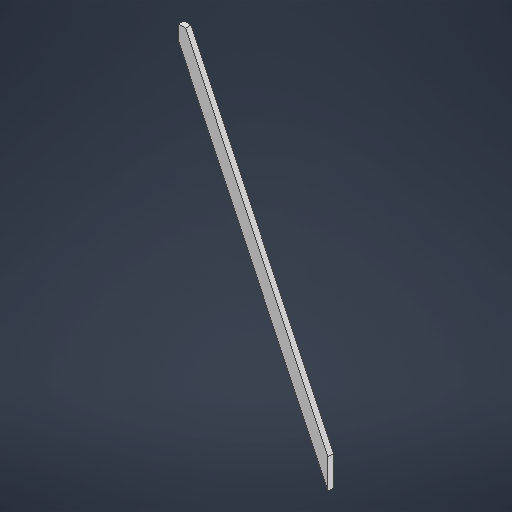
# Autodesk Inventor part: S_2x4x99.417
Saved by Autodesk Inventor 2026 (Build 300175000, 175)
## iProperties
Created: 2025-09-04
Part Number: S_2x4x99.417
Material: Generic
Document SubType Name: Modeling
Designer: trott
Density: 1 g/cm^3
Appearance: Default
Author: trott
Autodesk Inventor part; units mm, degrees
ref_plane "YZ Plane" through (0, 0, 0) normal (1, 0, 0) x (0, 1, 0)
ref_plane "XZ Plane" through (0, 0, 0) normal (0, 1, 0) x (-1, 0, 0)
ref_plane "XY Plane" through (0, 0, 0) normal (0, 0, 1) x (1, 0, 0)
sketch "Sketch1" plane through (0, 0, 0) normal (0, 0, 1) x (1, 0, 0)
  line L0 (-520.7, -2197.1) -> (520.7, -2197.1)
  line L1 (520.7, -2197.1) -> (520.7, 2197.1)
  line L2 (520.7, 2197.1) -> (-520.7, 2197.1)
  line L3 (-520.7, 2197.1) -> (-520.7, -2197.1)
  line L4 (-520.7, -2197.1) -> (520.7, 2197.1) construction
  line L5 (520.7, -2197.1) -> (-520.7, 2197.1) construction
  line L6 (-520.7, 0) -> (520.7, 0)
  line L7 (520.7, 0) -> (-520.7, -2197.1)
  line L8 (-480.5336, -2216.1384) -> (-560.8664, -2178.0616)
  line L9 (560.8664, -19.0384) -> (480.5336, 19.0384)
  line L10 (480.5336, 19.0384) -> (-560.8664, -2178.0616)
  line L11 (-480.5336, -2216.1384) -> (560.8664, -19.0384)
  line L12 (480.5336, 19.0384) -> (520.7, 103.7798)
  line L13 (-520.7, 2197.1) -> (520.7, -2197.1) construction
  line L14 (520.7, 0) -> (-520.7, 2197.1)
  line L15 (-480.5336, 2216.1384) -> (-560.8664, 2178.0616)
  line L16 (560.8664, 19.0384) -> (480.5336, -19.0384)
  line L17 (480.5336, -19.0384) -> (-560.8664, 2178.0616)
  line L18 (-480.5336, 2216.1384) -> (560.8664, 19.0384)
  line L19 (480.5336, -19.0384) -> (520.7, -103.7798)
  point P0 (0, 0)
  point P1 (-471.5096, 2197.1)
  point P2 (-520.7, 2093.3202)
  point P3 (520.7, -103.7798)
  point P4 (520.7, -103.7798)
  point P5 (471.5096, 0)
  point P6 (-520.7, -2093.3202)
  point P7 (-471.5096, -2197.1)
  dimension "d0" = 1041.4
  dimension "d1" = 4394.2
  dimension "d3" = 88.9
  dimension "d4" = 88.9
  constraints: 40 end point, 6 midpoint, 5 symmetric about line, 3 perpendicular, 3 point on line, 2 parallel, 1 horizontal
  measures "d0" distance of L2.end L1.end
  measures "d1" distance of L0.end L1.end
  measures "d3" distance of L8.start L8.end
  measures "d4" distance of L9.start L9.end
extrude "Extrusion1" add sketch "Sketch1" along normal blind 38.1 contours L19 L16 L7 | L7 L1 L19 | L10 L9 L6 | L17 L3 L14 L12 L10 | L6 L16 L17 | L14 L12 L1 | L9 L12 L14 | L12 L14 L2 L18
body "Solid1"
